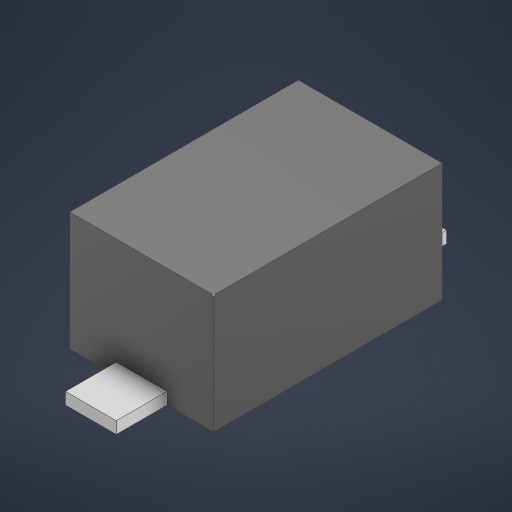
# Autodesk Inventor part: sod-123-model
Saved by Autodesk Inventor 2024.2 (Build 282272000, 272)
## iProperties
Created: 2024-08-08
Part Number: sod-123-model
Material: Generic
Document SubType Name: Modeling
Designer: Moe
Density: 1 g/cm^3
Appearance: Default
Author: Moe
Autodesk Inventor part; units mm, degrees
ref_plane "YZ Plane" through (0, 0, 0) normal (1, 0, 0) x (0, 1, 0)
ref_plane "XZ Plane" through (0, 0, 0) normal (0, 1, 0) x (-1, 0, 0)
ref_plane "XY Plane" through (0, 0, 0) normal (0, 0, 1) x (1, 0, 0)
sketch "Sketch1" plane through (0, 0, 0) normal (0, 1, 0) x (-1, 0, 0)
  line L0 (0, 0) -> (1.7, 0)
  line L1 (1.7, 0) -> (1.7, -2.7)
  line L2 (1.7, -2.7) -> (0, -2.7)
  line L3 (0, -2.7) -> (0, 0)
  dimension "d0" = 1.7
  dimension "d1" = 2.7
  constraints: 8 end point, 2 parallel, 1 horizontal, 1 perpendicular
  measures "d0" distance of L1.end L2.end
  measures "d1" distance of L0.end L1.end
extrude "Extrusion1" add sketch "Sketch1" along normal blind 1.4
sketch "Sketch2" plane through (-1.7, 0, 0) normal (0, 0, 1) x (1, 0, 0)
  line L0 (1.7, 0) -> (0, 0) projected
  line L1 (0.55, 0) -> (1.15, 0)
  line L2 (1.15, 0) -> (1.15, 0.14)
  line L3 (1.15, 0.14) -> (0.55, 0.14)
  line L4 (0.55, 0.14) -> (0.55, 0)
  line L5 (1.7, 0) -> (1.7, 1.4) projected
  dimension "d4" = 0.6
  dimension "d5" = 0.14
  dimension "d6" = 0.55
  constraints: 8 end point, 2 parallel, 1 horizontal, 1 perpendicular, 1 point on line
  measures "d4" distance of L3.end L2.end
  measures "d5" distance of L1.end L2.end
  measures "d6" distance between parallel lines of L5 L2
extrude "Extrusion2" add sketch "Sketch2" along normal blind 0.6
sketch "Sketch3" plane through (0, 0, -2.7) normal (0, 0, -1) x (-1, 0, 0)
  line L0 (0.55, 0) -> (1.15, 0)
  line L1 (1.15, 0) -> (1.15, 0.14)
  line L2 (1.15, 0.14) -> (0.55, 0.14)
  line L3 (0.55, 0.14) -> (0.55, 0)
  line L4 (1.7, 0) -> (1.7, 1.4) projected
  line L5 (0, 1.4) -> (1.7, 1.4) projected
  point P0 (0, 0)
  dimension "d9" = 0.6
  dimension "d10" = 0.14
  dimension "d11" = 0.55
  dimension "d12" = 1.4
  constraints: 8 end point, 2 parallel, 1 horizontal, 1 perpendicular
  measures "d9" distance of L2.end L1.end
  measures "d10" distance of L0.end L1.end
  measures "d11" distance between parallel lines of L4 L1
  measures "d12" distance between parallel lines of L5 L0
extrude "Extrusion3" add sketch "Sketch3" along normal blind 0.6
sketch "Sketch4" plane through (0, 1.4, 0) normal (0, 1, 0) x (1, 0, 0)
  point P0 (0, 0)
body "Solid1"
